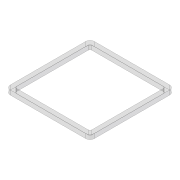
# Autodesk Inventor part: Adult fly trap middle
Saved by Autodesk Inventor 2020 (Build 240168000, 168)
## iProperties
Created: 2020-09-12
Part Number: Adult fly trap middle
Material: Generic
Document SubType Name: Modeling
Designer: ferrerx
Density: 1 g/cm^3
Appearance: Clear - Light
Author: ferrerx
Autodesk Inventor part; units mm, degrees
ref_plane "YZ Plane" through (0, 0, 0) normal (1, 0, 0) x (0, 1, 0)
ref_plane "XZ Plane" through (0, 0, 0) normal (0, 1, 0) x (-1, 0, 0)
ref_plane "XY Plane" through (0, 0, 0) normal (0, 0, 1) x (1, 0, 0)
sketch "Sketch1" plane through (0, 0, 0) normal (0, 1, 0) x (-1, 0, 0)
  line L0 (0, 0) -> (95, 0)
  line L1 (95, 0) -> (95, -95)
  line L2 (95, -95) -> (0, -95)
  line L3 (0, -95) -> (0, 0)
  dimension "d0" = 95
  dimension "d1" = 95
  constraints: 8 end point, 2 parallel, 1 horizontal, 1 perpendicular
  measures "d0" distance of L1.end L2.end
  measures "d1" distance of L2.end L0.start
extrude "Extrusion1" add sketch "Sketch1" along normal blind 5
sketch "Sketch2" plane through (0, 5, 0) normal (0, 1, 0) x (1, 0, 0)
  line L0 (-90, 5) -> (-5, 5)
  line L1 (-5, 5) -> (-5, 90)
  line L2 (-5, 90) -> (-90, 90)
  line L3 (-90, 90) -> (-90, 5)
  line L4 (0, 95) -> (-95, 95) projected
  line L5 (-95, 95) -> (-95, 0) projected
  line L6 (-95, 0) -> (0, 0) projected
  line L7 (0, 0) -> (0, 95) projected
  dimension "d4" = 5
  dimension "d5" = 5
  dimension "d6" = 5
  dimension "d7" = 5
  constraints: 8 end point, 2 parallel, 1 horizontal, 1 perpendicular
  measures "d4" distance between parallel lines of L4 L2
  measures "d5" distance between parallel lines of L5 L3
  measures "d6" distance between parallel lines of L6 L0
  measures "d7" distance between parallel lines of L7 L1
extrude "Extrusion2" cut sketch "Sketch2" against normal blind 5 contours L3 L2 L1 L0
fillet "Fillet1" radius 5 4 edges at (-95, 2.5, -95) (0, 2.5, 0) (0, 2.5, -95) (-95, 2.5, 0)
sketch "Sketch3" plane through (0, 5, 0) normal (0, 1, 0) x (1, 0, 0)
  line L0 (-92.5, 92.5) -> (-2.5, 92.5) construction
  line L1 (-2.5, 92.5) -> (-2.5, 2.5) construction
  line L2 (-2.5, 2.5) -> (-92.5, 2.5) construction
  line L3 (-92.5, 2.5) -> (-92.5, 92.5) construction
  line L4 (0, 5) -> (0, 90) projected
  line L5 (-5, 95) -> (-90, 95) projected
  line L6 (-95, 90) -> (-95, 5) projected
  line L7 (-90, 0) -> (-5, 0) projected
  point P0 (0, 0)
  dimension "d11" = 2.5
  dimension "d12" = 2.5
  dimension "d13" = 2.5
  dimension "d14" = 2.5
  constraints: 8 end point, 2 parallel, 1 horizontal, 1 perpendicular
  measures "d11" distance between parallel lines of L4 L1
  measures "d12" distance between parallel lines of L5 L0
  measures "d13" distance between parallel lines of L6 L3
  measures "d14" distance between parallel lines of L7 L2
fillet "Fillet2" radius 2 4 edges at (-90, 2.5, -90) (-5, 2.5, -90) (-5, 2.5, -5) (-90, 2.5, -5)
body "Solid1"
